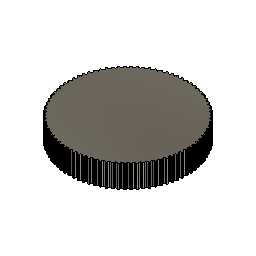
gear_84z (Autodesk Fusion 360 design; units mm, degrees)
Autodesk Fusion 360 part; units mm, degrees
sketch "Sketch1" plane through (0, 0, 0) normal (0, 0, 1) x (1, 0, 0) in component "gt2 pulley"
  circle A0 centre (0, 0) radius 26.738 construction
  circle A1 centre (0, 0) radius 25.734 construction
  line L0 (0, 0) -> (0, 26.738) construction
  line L1 (0, 0) -> (0.9998, 26.7193) construction
  line L2 (0, 0) -> (1.4047, 26.7011) construction
  circle A2 centre (0, 0) radius 26.484 construction
  arc A3 (0.3963, 26.3478) -> (0.4737, 26.0501) centre (1.3913, 26.4475) ccw
  circle A4 centre (0, 0) radius 26.334 construction
  arc A5 (0.2484, 26.4829) -> (0, 26.484) centre (0, 0) ccw
  arc A6 (0.3963, 26.3478) -> (0.2484, 26.4829) centre (0.2471, 26.3329) ccw
  arc A7 (0.4737, 26.0501) -> (0.9622, 25.716) centre (0.983, 26.2706) ccw
  arc A8 (0, 26.484) -> (-0.2484, 26.4829) centre (0, 0) ccw
  arc A9 (-0.2484, 26.4829) -> (-0.3963, 26.3478) centre (-0.2471, 26.3329) ccw
  arc A10 (-0.4737, 26.0501) -> (-0.3963, 26.3478) centre (-1.3913, 26.4475) ccw
  arc A11 (-0.9622, 25.716) -> (-0.4737, 26.0501) centre (-0.983, 26.2706) ccw
  arc A12 (0.9622, 25.716) -> (-0.9622, 25.716) centre (0, 0) ccw
  point P0 (1.3913, 26.4475)
  point P1 (0, 26.484)
  dimension "d18" = 53.4761
  dimension "d19" = 2.143
  dimension "d22" = 1.004
  dimension "d24" = 0.75
  dimension "d26" = 1
  dimension "d27" = 0.15
  dimension "d28" = 0.15
  dimension "d47" = 0.555
  dimension "d52" = 3.812
  constraint coincident A0.centre A1.centre
  constraint coincident A0 L0.end
  constraint vertical L0
  constraint coincident A0 L1.end
  constraint coincident A0 L2.end
  constraint concentric A1 A2
  constraint coincident A1 A7.end
  constraint coincident L1 A7.end
  constraint coincident A2 P0
  constraint coincident L2 P0
  constraint coincident P0 A3.centre
  constraint coincident A2 P1
  constraint coincident L0 P1
  constraint concentric A2 A4
  constraint coincident P1 A5.end
  constraint coincident A4 A6.centre
  constraint coincident A3.start A6.start
  constraint tangent A3 A6
  constraint tangent A3 A7
  constraint symmetric L0 A7.end A11.start
  constraint symmetric L0 A3.start A9.end
  constraint symmetric L0 A3.end A10.start
  constraint symmetric L0 A3 A10
  constraint symmetric L0 A5.start A8.end
  constraint symmetric L0 P1 A5.end
  constraint symmetric L0 A5 A8
  constraint symmetric L0 A6 A9
  constraint symmetric L0 A7 A11
  constraint coincident A1 A11.start
  constraint tangent A1 A7
  constraint coincident L1 A7.centre
  measures "d18" diameter of A0
  measures "d19" angle of L0 L1
  measures "d22" distance of A0 A1
  measures "d24" distance of A1 A2
  measures "d26" radius of A3
  measures "d27" distance of A2 A4
  measures "d28" radius of A6
  measures "d47" radius of A7
extrude "Extrude1" add sketch "Sketch1" along normal blind 10 makes body 1
pattern_circular "C-Pattern1" count 84 over 360 about axis through (0, 0, 1.75) along (0, 0, 1) of bodies 1 makes body 2 at (-1.1759, 25.7071, 3.3333) makes body 3 at (-4.3633, 25.3614, 6.6667) makes body 4 at (-4.9942, 25.2448, 3.3333) makes body 5 at (-6.8668, 24.801, 3.3333) makes body 6 at (-10.0944, 23.6716, 6.6667) makes body 7 at (-11.2618, 23.139, 6.6667) makes body 8 at (-12.9595, 22.2327, 6.6667) makes body 9 at (-14.5847, 21.2021, 6.6667) makes body 10 at (-16.6232, 19.6445, 6.6667) makes body 11 at (-18.0448, 18.3474, 6.6667) makes body 12 at (-18.9369, 17.4251, 6.6667) makes body 13 at (-19.6445, 16.6233, 3.3333) makes body 14 at (-20.8318, 15.1088, 3.3333) makes body 15 at (-22.6511, 12.2134, 6.6667) makes body 16 at (-23.5005, 10.4866, 6.6667) makes body 17 at (-24.2184, 8.701, 6.6667) makes body 18 at (-24.8009, 6.8669, 6.6667) makes body 19 at (-24.9117, 6.4536, 6.6667) makes body 20 at (-25.5474, 3.0938, 6.6667) makes body 21 at (-25.6698, 1.8165, 6.6667) makes body 22 at (-25.7338, -0.1069, 6.6667) makes body 23 at (-25.7071, -1.1759, 3.3333) makes body 24 at (-25.4305, -3.9411, 6.6667) makes body 25 at (-25.0648, -5.8305, 6.6667) makes body 26 at (-24.3597, -8.2972, 6.6667) makes body 27 at (-24.2184, -8.701, 3.3333) makes body 28 at (-23.5005, -10.4865, 3.3333) makes body 29 at (-21.9027, -13.5097, 6.6667) makes body 30 at (-21.6751, -13.8719, 3.3333) makes body 31 at (-19.6445, -16.6232, 6.6667) makes body 32 at (-19.3655, -16.9475, 3.3333) makes body 33 at (-16.9476, -19.3654, 6.6667) makes body 34 at (-16.6233, -19.6445, 3.3333) makes body 35 at (-15.1088, -20.8318, 3.3333) makes body 36 at (-12.7743, -22.3396, 6.6667) makes body 37 at (-11.8352, -22.851, 3.3333) makes body 38 at (-10.0945, -23.6716, 3.3333) makes body 39 at (-7.483, -24.622, 6.6667) makes body 40 at (-4.9943, -25.2447, 6.6667) makes body 41 at (-3.7297, -25.4623, 6.6667) makes body 42 at (-1.8165, -25.6698, 6.6667) makes body 43 at (0.1069, -25.7338, 6.6667) makes body 44 at (1.1759, -25.7071, 3.3333) makes body 45 at (4.3633, -25.3614, 6.6667) makes body 46 at (4.9942, -25.2448, 3.3333) makes body 47 at (6.8668, -24.801, 3.3333) makes body 48 at (9.5011, -23.9159, 6.6667) makes body 49 at (11.2618, -23.139, 6.6667) makes body 50 at (12.2134, -22.6511, 3.3333) makes body 51 at (14.5847, -21.2021, 6.6667) makes body 52 at (16.6232, -19.6445, 6.6667) makes body 53 at (17.5818, -18.7915, 6.6667) makes body 54 at (19.3654, -16.9476, 6.6667) makes body 55 at (19.6445, -16.6233, 3.3333) makes body 56 at (21.6751, -13.872, 6.6667) makes body 57 at (22.6511, -12.2134, 6.6667) makes body 58 at (23.5005, -10.4866, 6.6667) makes body 59 at (23.994, -9.3021, 6.6667) makes body 60 at (24.622, -7.483, 6.6667) makes body 61 at (24.9117, -6.4536, 6.6667) makes body 62 at (25.4623, -3.7297, 6.6667) makes body 63 at (25.6698, -1.8165, 6.6667) makes body 64 at (25.7338, 0.1069, 6.6667) makes body 65 at (25.7071, 1.1759, 3.3333) makes body 66 at (25.5474, 3.0937, 3.3333) makes body 67 at (25.2448, 4.9942, 3.3333) makes body 68 at (24.801, 6.8668, 3.3333) makes body 69 at (23.6716, 10.0944, 6.6667) makes body 70 at (23.5005, 10.4865, 3.3333) makes body 71 at (22.6511, 12.2134, 3.3333) makes body 72 at (21.2021, 14.5847, 6.6667) makes body 73 at (19.6445, 16.6232, 6.6667) makes body 74 at (18.7915, 17.5818, 6.6667) makes body 75 at (18.0449, 18.3473, 3.3333) makes body 76 at (16.6233, 19.6445, 3.3333) makes body 77 at (15.1088, 20.8318, 3.3333) makes body 78 at (12.2134, 22.6511, 6.6667) makes body 79 at (11.8352, 22.851, 3.3333) makes body 80 at (9.3021, 23.994, 6.6667) makes body 81 at (7.483, 24.622, 6.6667) makes body 82 at (6.4536, 24.9117, 6.6667) makes body 83 at (3.7297, 25.4623, 6.6667) makes body 84 at (1.8165, 25.6698, 6.6667)
sketch "Sketch2" plane through (0, 0, 10) normal (0, 0, 1) x (-1, 0, 0)
  arc A0 (-11.789, -23.5666) -> (-11.7143, -23.7525) centre (-11.648, -23.6179) ccw
  arc A1 (-11.7143, -23.7525) -> (-11.2667, -23.968) centre (0, 0) ccw
  arc A2 (-11.2667, -23.968) -> (-11.0748, -23.9105) centre (-11.2028, -23.8323) ccw
  arc A3 (-10.876, -23.6759) -> (-11.0748, -23.9105) centre (-10.2216, -24.432) ccw
  arc A4 (-10.2909, -23.5868) -> (-10.876, -23.6759) centre (-10.5128, -24.0955) ccw
  arc A5 (-12.0247, -22.7519) -> (-10.2909, -23.5868) centre (0, 0) ccw
  arc A6 (-11.7295, -23.2648) -> (-12.0247, -22.7519) centre (-12.284, -23.2425) ccw
  arc A7 (-11.789, -23.5666) -> (-11.7295, -23.2648) centre (-12.7287, -23.2247) ccw
  circle A8 centre (0, 0) radius 25.734
  constraint concentric A1 A8
extrude "Extrude2" add sketch "Sketch2" against normal blind 10 contours A5 A8 bodies 1 2 3 4 5 6 7 8 9 10 11 12 13 14 15 16 17 18 19 20 21 22 23 24 25 26 27 28 29 30 31 32 33 34 35 36 37 38 39 40 41 42 43 44 45 46 47 48 49 50 51 52 53 54 55 56 57 58 59 60 61 62 63 64 65 66 67 68 69 70 71 72 73 74 75 76 77 78 79 80 81 82 83 84
extrude "Extrude4" [suppressed] in component "gt2 pulley"
pattern_circular "C-Pattern7" [suppressed] in component "gt2 pulley"
extrude "Extrude3" [suppressed] in component "gt2 pulley"
pattern_circular "C-Pattern6" [suppressed] in component "gt2 pulley"
extrude "Extrude2'" [suppressed] in component "gt2 pulley"
pattern_circular "C-Pattern5" [suppressed] in component "gt2 pulley"
extrude "Extrude1'" [suppressed] in component "gt2 pulley"
pattern_circular "C-Pattern4" [suppressed] in component "gt2 pulley"
pattern_circular "C-Pattern3" [suppressed] in component "gt2 pulley"
pattern_circular "C-Pattern2" [suppressed] in component "gt2 pulley"
pattern_circular "C-Pattern1'" [suppressed] in component "gt2 pulley"
copy_body "Body->Comp1" [suppressed] in component "Component"
copy_body "Body->Comp2" [suppressed] in component "Component'"
copy_body "Body->Comp3" [suppressed] in component "Component''"
copy_body "Body->Comp4" [suppressed] in component "Component'''"
copy_body "Body->Comp5" [suppressed] in component "Component''''"
copy_body "Body->Comp6" [suppressed] in component "Component'''''"
copy_body "Body->Comp7" [suppressed] in component "Component''''''"
copy_body "Body->Comp8" [suppressed] in component "Component'''''''"
copy_body "Body->Comp9" [suppressed] in component "Component''''''''"
copy_body "Body->Comp10" [suppressed] in component "Component'''''''''"
copy_body "Body->Comp11" [suppressed] in component "Component''''''''''"
copy_body "Body->Comp12" [suppressed] in component "Component'''''''''''"
copy_body "Body->Comp13" [suppressed] in component "Component''''''''''''"
copy_body "Body->Comp14" [suppressed] in component "Component'''''''''''''"
copy_body "Body->Comp15" [suppressed] in component "Component''''''''''''''"
copy_body "Body->Comp16" [suppressed] in component "Component'''''''''''''''"
copy_body "Body->Comp17" [suppressed] in component "Component''''''''''''''''"
copy_body "Body->Comp18" [suppressed] in component "Component'''''''''''''''''"
copy_body "Body->Comp19" [suppressed] in component "Component''''''''''''''''''"
copy_body "Body->Comp20" [suppressed] in component "Component'''''''''''''''''''"
component "gt2 pulley" placed x (1, 0, 0) y (0, 1, 0) z (0, 0, 1) at (0, 0, 0)
equation "NumTeeth = 84" comment "min 20"
equation "ToothPitch = 2 mm"
equation "PullyDia = NumTeeth * ToothPitch / PI"
equation "ToothAng = ( ( 360 / NumTeeth ) * 1 deg )"
equation "TransOffsetAngle = ToothAng * 0.2"
equation "Sholulder_Radius = 0.15 mm"
equation "Root_Radius = 0.555 mm"
equation "TransRadius = 1 mm"
equation "ToolHeight = 0.75 mm"
equation "PLD = 0.254 mm"
equation "d18 = PullyDia"
equation "d19 = ToothAng / 2"
equation "d22 = PLD + ToolHeight"
equation "d24 = ToolHeight"
equation "d26 = TransRadius"
equation "d27 = Sholulder_Radius"
equation "d31 = NumTeeth"
equation "d33 = NumTeeth"
equation "d35 = NumTeeth"
equation "d37 = NumTeeth"
equation "d41 = NumTeeth"
equation "d45 = NumTeeth"
equation "d47 = Root_Radius"
equation "d50 = NumTeeth"
